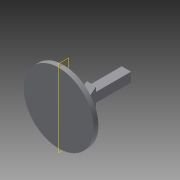
# Autodesk Inventor part: target
Saved by Autodesk Inventor 2013 (Build 170138000, 138)
## iProperties
Created: 2013-04-26
Part Number: target
Material: Generic
Document SubType Name: Modeling
Designer: otrab
Density: 1 g/cm^3
Author: otrab
Autodesk Inventor part; units mm, degrees
ref_plane "XZ Plane" through (0, 0, 0) normal (0, 1, 0) x (-1, 0, 0)
ref_plane "XY Plane" through (0, 0, 0) normal (0, 0, 1) x (1, 0, 0)
sketch "Sketch1" plane through (0, 0, 0) normal (0, 1, 0) x (-1, 0, 0)
  circle A0 centre (0, 0) radius 15
  circle A1 centre (0, 0) radius 12
  dimension "d0" = 30
  dimension "d2" = 24
  constraints: 2 centre point, 1 coincident
  measures "d0" diameter of A0
  measures "d2" diameter of A1
extrude "Extrusion1" add sketch "Sketch1" along normal blind 2
sketch "Sketch2" plane through (0, 0, 0) normal (0, -1, 0) x (1, 0, 0)
  circle A0 centre (0, 0) radius 12 projected
  circle A1 centre (0, 0) radius 15 projected
  circle A2 centre (0, 0) radius 5
  dimension "d5" = 10
  constraints: 1 centre point, 1 coincident
  measures "d5" diameter of A2
extrude "Extrusion2" add sketch "Sketch2" against normal blind 3 contours A0
sketch "Sketch3" plane through (0, 0, 0) normal (0, -1, 0) x (1, 0, 0)
  circle A0 centre (0, 0) radius 5 projected
extrude "Extrusion3" add sketch "Sketch3" against normal blind 4
ref_plane "Work Plane1" through (0, 0, 0) normal (1, 0, 0) x (0, 1, 0)
sketch "Sketch4" plane through (0, 0, 0) normal (1, 0, 0) x (0, 1, 0)
  line L0 (26.9981, 0) -> (26.9981, -2)
  line L1 (26.9981, -2) -> (11.9981, -2)
  line L2 (11.9981, -2) -> (11.9981, -4)
  line L3 (11.9981, -4) -> (7.1092, 0)
  line L4 (28.7393, 0) -> (4.7365, 0) construction
  line L5 (26.9981, 0) -> (26.9981, 2)
  line L6 (26.9981, 2) -> (11.9981, 2)
  line L7 (11.9981, 2) -> (11.9981, 4)
  line L8 (11.9981, 4) -> (7.1092, 0)
  point P0 (0, 0)
  dimension "d12" = 15
  dimension "d13" = 2
  constraints: 18 end point, 3 symmetric about line, 1 parallel, 1 perpendicular, 1 vertical
  measures "d12" distance of L0.end L1.end
  measures "d13" distance of L1.end L2.end
extrude "Extrusion4" add sketch "Sketch4" along normal blind 4
body "Solid1"
